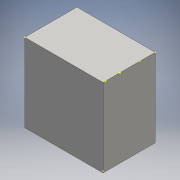
# Autodesk Inventor part: base
Saved by Autodesk Inventor 2016 (Build 200138000, 138)
## iProperties
Created: 2016-04-06
Part Number: base
Material: Genérico
Document SubType Name: Modeling
Designer: Usuario
Density: 1 g/cm^3
Appearance: Valor por defecto
Author: Usuario
Autodesk Inventor part; units mm, degrees
ref_plane "YZ Plane" through (0, 0, 0) normal (1, 0, 0) x (0, 1, 0)
ref_plane "XZ Plane" through (0, 0, 0) normal (0, 1, 0) x (-1, 0, 0)
ref_plane "XY Plane" through (0, 0, 0) normal (0, 0, 1) x (1, 0, 0)
sketch "Boceto1" plane through (0, 0, 0) normal (0, 1, 0) x (-1, 0, 0)
  point P0 (0, 0)
extrude "Extrusión1" [suppressed]
feature "Vaciado1" [suppressed]
sketch "Boceto2" plane through (0, 70, 0) normal (0, 1, 0) x (1, 0, 0)
  line L0 (-5, 5) -> (-5, 145) projected
  line L1 (-145, 145) -> (-145, 5) projected
  line L2 (-145, 5) -> (-5, 5) projected
  line L3 (-5, 145) -> (-145, 145) projected
  line L4 (-150, 0) -> (0, 0) projected
  circle A0 centre (-46.4922, 78) radius 12.5
  circle A1 centre (-46.4922, 78) radius 13.5
  constraints: 2 centre point, 2 coincident
hole "Agujero1" [suppressed]
sketch "Boceto3" plane through (0, 70, 0) normal (0, 1, 0) x (1, 0, 0)
  point P0 (0, 0)
sketch "Boceto4" plane through (0, 0, 0) normal (0, 1, 0) x (-1, 0, 0)
  point P0 (0, 0)
extrude "Extrusión2" [suppressed]
feature "Vaciado2" [suppressed]
sketch "Boceto5" plane through (0, 100, 0) normal (0, 1, 0) x (1, 0, 0)
  line L0 (0, 0) -> (0, 150) projected
  circle A0 centre (-46.5, 67.5) radius 14.5
  constraints: 1 centre point
extrude "Extrusión3" [suppressed]
sketch "Boceto6" plane through (0, 100, 0) normal (0, 1, 0) x (1, 0, 0)
  circle A0 centre (-46.5, 67.5) radius 12.5
  constraints: 1 centre point
extrude "Extrusión4" [suppressed]
sketch "Boceto7" plane through (-46.5, 31, -67.5) normal (0, -1, 0) x (1, 0, 0)
  point P0 (46.5, 67.5)
sketch "Boceto8" plane through (-46.5, 33, -67.5) normal (0, 1, 0) x (1, 0, 0)
  point P0 (46.5, -67.5)
sketch "Boceto9" plane through (0, 100, 0) normal (0, 1, 0) x (1, 0, 0)
  point P0 (0, 0)
sketch "Boceto10" plane through (0, 0, 0) normal (0, 1, 0) x (-1, 0, 0)
  line L0 (0, 0) -> (0, -150)
  line L1 (0, -150) -> (150, -150)
  line L2 (150, -150) -> (150, 0)
  line L3 (150, 0) -> (0, 0)
  constraints: 8 end point, 2 perpendicular, 1 vertical
extrude "Extrusión5" add sketch "Boceto10" along normal blind 100
shell "Vaciado3" thickness 3 removed faces 1 at (-150, 33.3333, -100)
sketch "Boceto11" plane through (0, 100, 0) normal (0, 1, 0) x (1, 0, 0)
  line L0 (-150, 0) -> (0, 0) projected
  line L1 (0, 0) -> (0, 150) projected
  circle A0 centre (-46.5, 67.5) radius 12.5002
  constraints: 1 centre point
extrude "Extrusión6" add sketch "Boceto11" against normal blind 4
sketch "Boceto12" plane through (0, 100, 0) normal (0, 1, 0) x (1, 0, 0)
  circle A0 centre (-46.5, 67.5) radius 12.5
  point P0 (0, 0)
  constraints: 1 centre point
extrude "Extrusión7" cut sketch "Boceto12" against normal blind 1
sketch "Boceto13" plane through (0, 100, 0) normal (0, 1, 0) x (1, 0, 0)
  point P0 (0, 0)
sketch "Boceto14" plane through (-46.5, 96, -67.5) normal (0, -1, 0) x (1, 0, 0)
  circle A0 centre (0, 0) radius 3.5
  point P0 (46.5, 67.5)
  constraints: 1 centre point
extrude "Extrusión8" cut sketch "Boceto14" against normal blind 3
sketch "Boceto15" plane through (-46.5, 99, -67.5) normal (0, 1, 0) x (1, 0, 0)
  circle A0 centre (0, -8.5) radius 1.5
  circle A1 centre (0, 8.5) radius 1.5
  point P0 (46.5, -67.5)
  constraints: 2 centre point
extrude "Extrusión9" cut sketch "Boceto15" against normal blind 3
sketch "Boceto16" plane through (-150, 0, -150) normal (-1, 0, 0) x (0, 0, 1)
  line L0 (3, 97) -> (147, 97) projected
  line L1 (4, 96) -> (146, 96)
  line L2 (147, 3) -> (3, 3) projected
  line L3 (4, 4) -> (4, 96)
  line L4 (146, 4) -> (4, 4)
  line L5 (146, 96) -> (146, 4)
  line L6 (3, 97) -> (147, 97)
  line L7 (147, 3) -> (147, 97) projected
  line L8 (147, 3) -> (3, 3)
  line L9 (3, 3) -> (3, 97) projected
  line L10 (3, 97) -> (3, 3)
  line L11 (147, 97) -> (147, 3)
  point P0 (150, 0)
  constraints: 16 end point, 2 collinear, 1 perpendicular, 1 vertical
sketch "Boceto17" plane through (-150, 3, -147) normal (0, 0, 1) x (1, 0, 0)
  point P0 (150, -3)
extrude "Extrusión10" add sketch "Boceto16" against normal blind 148
sketch "Boceto18" plane through (-46.5, 97, -67.5) normal (0, 1, 0) x (1, 0, 0)
  circle A0 centre (0, 0) radius 3.5
  point P0 (46.5, -67.5)
  constraints: 1 centre point
extrude "Extrusión11" cut sketch "Boceto18" against normal blind 1
sketch "Boceto19" plane through (-150, 0, -150) normal (-1, 0, 0) x (0, 0, 1)
  point P0 (150, 0)
sketch "Boceto20" plane through (-46.5, 97, -76) normal (0, 1, 0) x (1, 0, 0)
  circle A0 centre (0, 0) radius 1.5 projected
  circle A1 centre (0, 0) radius 1.5
  circle A2 centre (0, -17) radius 1.5
  point P0 (46.5, -76)
  constraints: 2 centre point, 1 coincident
extrude "Extrusión12" cut sketch "Boceto20" against normal blind 1
sketch "Boceto21" plane through (-150, 0, -150) normal (-1, 0, 0) x (0, 0, 1)
  point P0 (150, 0)
sketch "Boceto22" plane through (-150, 4, -4) normal (0, 1, 0) x (1, 0, 0)
  point P0 (150, -4)
  point P1 (0, 142)
sketch "Boceto23" plane through (0, 0, 0) normal (0, -1, 0) x (1, 0, 0)
  point P0 (0, 0)
extrude "Extrusión13" [suppressed]
sketch "Boceto24" plane through (0, 5, 0) normal (0, 1, 0) x (1, 0, 0)
  point P0 (0, 0)
sketch "Boceto25" plane through (0, 0, 0) normal (0, -1, 0) x (1, 0, 0)
  line L0 (-150, -146) -> (-150, -4) projected
  line L1 (-150, -146) -> (-45.9, -146)
  line L2 (-45.9, -146) -> (-45.9, -90.1)
  line L3 (-45.9, -90.1) -> (-150, -90.1)
  line L4 (-150, -146) -> (-150, -145)
  line L5 (-149, -145) -> (-46.9, -145)
  line L6 (-45.9, -146) -> (-46.9, -146)
  line L7 (-46.9, -145) -> (-46.9, -91.1)
  line L8 (-45.9, -90.1) -> (-45.9, -91.1)
  line L9 (-46.9, -91.1) -> (-149, -91.1)
  line L10 (-150, -90.1) -> (-149, -90.1)
  line L11 (-149, -145) -> (-149, -144)
  line L12 (-149, -144) -> (-150, -144)
  line L13 (-149, -91.1) -> (-149, -92.1)
  line L14 (-149, -92.1) -> (-150, -92.1)
  line L15 (-149, -91.1) -> (-149, -92.1)
  line L16 (-149, -144) -> (-149, -145)
  line L17 (-150, -146) -> (-150, -144)
  line L18 (-150, -92.1) -> (-150, -90.1)
  point P0 (0, 0)
  constraints: 36 end point, 8 perpendicular, 7 point on line
extrude "Extrusión14" add sketch "Boceto25" against normal blind 5 contours L0 L12 L11 L5 L7 L9 L13 L14 L3 L2 L1
sketch "Boceto26" plane through (-150, 4, -4) normal (0, 1, 0) x (1, 0, 0)
  line L0 (0, 0) -> (147, 0) projected
  line L1 (0, 0) -> (46, 0)
  line L2 (46, 0) -> (46, 46)
  line L3 (46, 46) -> (0, 46)
  line L4 (0, 0) -> (0, 86.1) projected
  line L5 (46, 46) -> (45, 46)
  line L6 (46, 46) -> (46, 45)
  line L7 (45, 45) -> (1, 45)
  line L8 (0, 46) -> (1, 46)
  line L9 (0, 0) -> (0, 1)
  line L10 (46, 46) -> (45, 46)
  line L11 (45, 45) -> (45, 1)
  line L12 (1, 1) -> (45, 1)
  line L13 (1, 45) -> (1, 44)
  line L14 (1, 44) -> (0, 44)
  line L15 (1, 1) -> (1, 2)
  line L16 (1, 2) -> (0, 2)
  line L17 (0, 46) -> (0, 44)
  line L18 (0, 2) -> (0, 0)
  line L19 (1, 45) -> (1, 44)
  line L20 (1, 2) -> (1, 1)
  point P0 (150, -4)
  constraints: 38 end point, 5 point on line, 2 vertical, 1 collinear, 1 horizontal, 1 midpoint, 1 perpendicular
extrude "Extrusión15" add sketch "Boceto26" along normal blind 1 contours L4 L16 L15 L12 L11 L7 L13 L14 L3 L2 L0
